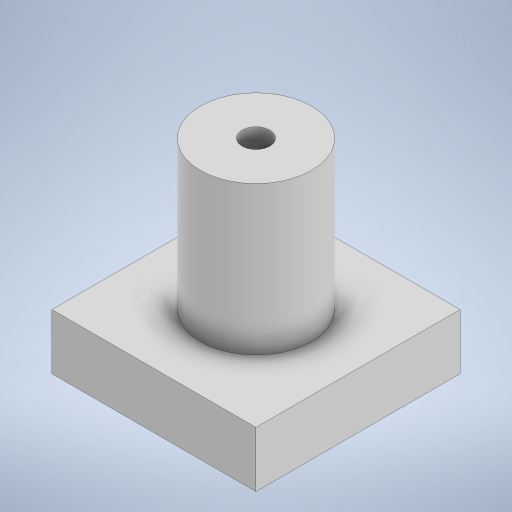
# Autodesk Inventor part: oparil
Saved by Autodesk Inventor 2024 (Build 280153000, 153)
## iProperties
Created: 2024-05-15
Part Number: oparil
Material: Všeobecné
Document SubType Name: Modeling
Designer: eliasla
Density: 1 g/cm^3
Appearance: Výchozí
Author: eliasla
Autodesk Inventor part; units mm, degrees
ref_plane "YZ Plane" through (0, 0, 0) normal (1, 0, 0) x (0, 1, 0)
ref_plane "XZ Plane" through (0, 0, 0) normal (0, 1, 0) x (-1, 0, 0)
ref_plane "XY Plane" through (0, 0, 0) normal (0, 0, 1) x (1, 0, 0)
sketch "Náčrt1" plane through (0, 0, 0) normal (0, 0, 1) x (1, 0, 0)
  line L0 (0, 0) -> (11, 0)
  line L1 (11, 0) -> (11, 11)
  line L2 (11, 11) -> (0, 11)
  line L3 (0, 11) -> (0, 0)
  dimension "d0" = 11
  dimension "d1" = 11
  constraints: 8 end point, 2 parallel, 1 horizontal, 1 perpendicular
  measures "d0" distance of L0.end L1.end
  measures "d1" distance of L1.end L2.end
extrude "Vysunutí1" add sketch "Náčrt1" along normal blind 3
sketch "Náčrt2" plane through (0, 0, 3) normal (0, 0, 1) x (1, 0, 0)
  circle A0 centre (5.5, 5.5) radius 3
  line L0 (0, 0) -> (11, 0) projected
  point P0 (5.5, 0)
  dimension "d4" = 6
  dimension "d5" = 5.5
  constraints: 1 centre point, 1 midpoint
  measures "d4" diameter of A0
  measures "d5" distance of A0.centre point (5.5, 0)
extrude "Vysunutí2" add sketch "Náčrt2" along normal blind 8
sketch "Náčrt3" plane through (5.5, 5.5, 11) normal (0, 0, 1) x (1, 0, 0)
  circle A0 centre (0, 0) radius 0.75
  point P0 (-5.5, -5.5)
  dimension "d8" = 1.5
  constraints: 1 centre point
  measures "d8" diameter of A0
extrude "Vysunutí3" cut sketch "Náčrt3" against normal through all
